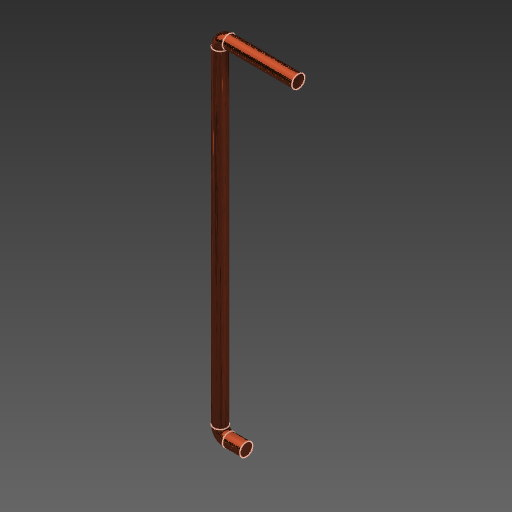
# Autodesk Inventor part: TopPipeStraight
Saved by Autodesk Inventor 2020.4 (Build 244396010, 396A)
## iProperties
Created: 2022-09-12
Part Number: TopPipeStraight
Material: Copper, Cast
Document SubType Name: Modeling
Designer: Val
Density: 8.94 g/cm^3
Appearance: Copper - Satin
Author: Val
Autodesk Inventor part; units mm, degrees
ref_plane "YZ Plane" through (0, 0, 0) normal (1, 0, 0) x (0, 1, 0)
ref_plane "XZ Plane" through (0, 0, 0) normal (0, 1, 0) x (-1, 0, 0)
ref_plane "XY Plane" through (0, 0, 0) normal (0, 0, 1) x (1, 0, 0)
sketch "PipeSide" plane through (0, 0, 0) normal (0, 0, 1) x (1, 0, 0)
  line L0 (-25.4, 328.0833) -> (-25.4, 8.4667)
  line L1 (-16.9333, 0) -> (0, 0)
  line L2 (-16.9333, 336.55) -> (50.8, 336.55)
  arc A0 (-25.4, 8.4667) -> (-16.9333, 0) centre (-16.9333, 8.4667) ccw
  arc A1 (-16.9333, 336.55) -> (-25.4, 328.0833) centre (-16.9333, 328.0833) ccw
  point P0 (-25.4, 336.55)
  point P1 (-25.4, 0)
  point P2 (75.9666, 233.9144)
  point P3 (76.9893, 233.9144)
  dimension "d1" = 76.2
  dimension "d2" = 336.55
  dimension "d3" = 25.4
  dimension "d19" = 8.4667
  constraints: 6 end point, 4 point on circle, 4 point on line, 4 tangent, 2 centre point, 2 perpendicular, 1 coincident, 1 equal radius, 1 vertical
  measures "d1" distance of point (-25.4, 336.55) L2.end
  measures "d2" distance of point (-25.4, 336.55) point (-25.4, 0)
  measures "d3" distance of point (-25.4, 0) L1.end
  measures "d19" radius of A0
sketch "PipeProfile" plane through (0, 0, 0) normal (1, 0, 0) x (0, 1, 0)
  circle A0 centre (0, 0) radius 6.35
  dimension "d18" = 12.7
  constraints: 1 centre point, 1 coincident
  measures "d18" diameter of A0
sweep "Sweep4" add profiles "PipeProfile" path "PipeSide"
body "Solid6"
